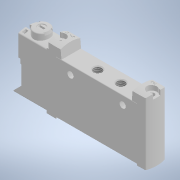
# Autodesk Inventor part: 564212 VUVG-L-10-M52-M-T-M5--1H2--L-W1---(G)
Saved by Autodesk Inventor 2021 (Build 250183000, 183)
## iProperties
Created: 2026-04-25
Part Number: 564212 VUVG-L-10-M52-M-T-M5--1H2--L-W1---(G)
Material: Generic
Catalog Web Link: www.3dfindit.com
Description: VUVG-(G)-Directional control valves for standard applications
Vendor: FESTO
Document SubType Name: Modeling
Designer: psAdmin
Manufacturer: FESTO
Mass: 17.6893 g
Surface Area: 76.999 cm^2
Volume: 17.6893 cm^3
Density: 1 g/cm^3
Appearance: PSOLRGB-176-176-176
Category: PARTsolutions
Company: FESTO
Title: 564212 VUVG-L-10-M52-M-T-M5--1H2--L-W1---(G)
Author: Cadenas PARTsolutions
Comments: Directional control valves for standard applications
PSOL_IDENT_0: {$CADENAS_DATA/23d-libs/festo/parts/v/vuvg/parts/vuvg_gehause.prj},283 {VTYP=3D},{NB=564212 VUVG-L-1
PSOL_IDENT_1: 0-M52-M-T-M5--1H2--L-W1---(G)},{LINA=564212 VUVG-L-10-M52-M-T-M5--1H2--L-W1---(G)},{NN=VUVG-(G)},{DA
PSOL_IDENT_2: TE=05.06.2024 09:23:06},{GEOMDATE=05.06.2024 09:22:54},{VERSION=},{LINEID=10},{WBVAR=VA,KP,BG,VF,RS,
PSOL_IDENT_3: SZ,HHB,PA,EL,NS,EA,SBS,ANZ,EZV,KUP,ZUL},{WBNUMERIC=}  {NB=564212 VUVG-L-10-M52-M-T-M5--1H2--L-W1---(
PSOL_IDENT_4: G)},{LINA=564212 VUVG-L-10-M52-M-T-M5--1H2--L-W1---(G)},{KT=DUMMY},{TNR=564212},{TYP=VUVG},{VA=L},{K
PSOL_IDENT_5: P=-},{BG=10},{VF=M52},{RS=M},{SZ=-},{HHB=T},{PA=M5},{EL=-},{NS=1},{EA=H2},{SBS=-},{ANZ=L},{EZV=W1},{
PSOL_IDENT_6: KUP=-},{ZUL=-},{KZU=-},{L=42},{L1=7.5},{L2=41.62},{H1=1.2},{THREAD=5},{VERS=1},{ASP=1},{CODE=},{SCAL
PSOL_IDENT_7: E=0.5},{ZUL1=},{KZU1=},{ZULT='-'},{KUP1=},{KUPW='-','F1A'}
NB: 564212 VUVG-L-10-M52-M-T-M5--1H2--L-W1---(G)
NN: VUVG-(G)
NT: Directional control valves for standard applications
NBSYN: $TNR. $TYP.-$VA.$KP.$BG.-$VF.-$RS.$SZ.$HHB.-$PA.$EL.-$NS.$EA.-$SBS.$ANZ.-$EZV.$KUP1.$ZUL1.$KZU1.---(G)
LINA: 564212 VUVG-L-10-M52-M-T-M5--1H2--L-W1---(G)
CATALOG: Festo
TNR: 564212
TYP: VUVG
VA: L
KP: -
BG: 10
VF: M52
RS: M
SZ: -
HHB: T
PA: M5
EL: -
NS: 1
EA: H2
SBS: -
ANZ: L
EZV: W1
KUP: -
ZUL: -
KUPW: '-','F1A'
SUPPLIER: FESTO
ARTICLENO: 564212 VUVG-L-10-M52-M-T-M5--1H2--L-W1---(G)
BOMINFO: 564212 VUVG-L-10-M52-M-T-M5--1H2--L-W1---(G)
CREATOR: CADENAS GmbH
Autodesk Inventor part; units mm, degrees
sketch "Sketch_53" plane through (0, 0, 0) normal (1, 0, 0) x (0, 1, 0)
  line L0 (26.7, 5.1) -> (0, 5.1)
  line L1 (0, 5.1) -> (0, -5.1)
  line L2 (0, -5.1) -> (26.7, -5.1)
  arc A0 (26.7, -5.1) -> (27, -4.8) centre (26.7, -4.8) ccw
  line L3 (27, -4.8) -> (27, 4.8)
  arc A1 (27, 4.8) -> (26.7, 5.1) centre (26.7, 4.8) ccw
  constraints: 8 end point, 4 point on circle, 2 centre point
extrude "Extrusion1" add sketch "Sketch_53" along normal mid plane 42
sketch "Sketch_54" plane through (0, 0, 0) normal (0, 0, 1) x (1, 0, 0)
  circle A0 centre (13.5, 22.6) radius 1.6
  constraints: 1 centre point
extrude "Extrusion2" cut sketch "Sketch_54" along normal mid plane 12
sketch "Sketch_55" plane through (0, 0, 0) normal (0, 0, 1) x (1, 0, 0)
  circle A0 centre (-13.5, 22.6) radius 1.6
  constraints: 1 centre point
extrude "Extrusion3" cut sketch "Sketch_55" along normal mid plane 12
sketch "Sketch4" plane through (-21, 0, -5.1) normal (0, -1, 0) x (1, 0, 0)
  point P0 (33.5, 5.1)
hole "Hole1" at (12.5, 0, 0) direction (0, 1, 0) diameter 4.134 depth 13.5 countersink diameter 5 countersink angle 90 thread size "M5x0.8" class "6H" standard "ISO Metric profile"
sketch "Sketch5" plane through (-21, 0, -5.1) normal (0, -1, 0) x (1, 0, 0)
  point P0 (22.5, 5.1)
hole "Hole2" at (1.5, 0, 0) direction (0, 1, 0) diameter 4.134 depth 18.8 tip angle 120 countersink diameter 5 countersink angle 90 thread size "M5x0.8" class "6H" standard "ISO Metric profile"
sketch "Sketch6" plane through (-21, 0, -5.1) normal (0, -1, 0) x (1, 0, 0)
  point P0 (11.5, 5.1)
hole "Hole3" at (-9.5, 0, 0) direction (0, 1, 0) diameter 4.134 depth 13.5 countersink diameter 5 countersink angle 90 thread size "M5x0.8" class "6H" standard "ISO Metric profile"
sketch "Sketch7" plane through (-21, 27, 4.8) normal (0, 1, 0) x (1, 0, 0)
  point P0 (16.5, 4.8)
hole "Hole4" at (-4.5, 27, 0) direction (0, -1, 0) diameter 4.134 depth 6.6 countersink diameter 5 countersink angle 90 thread size "M5x0.8" class "6H" standard "ISO Metric profile"
sketch "Sketch8" plane through (-21, 27, 4.8) normal (0, 1, 0) x (1, 0, 0)
  point P0 (28.5, 4.8)
hole "Hole5" at (7.5, 27, 0) direction (0, -1, 0) diameter 4.134 depth 6.6 countersink diameter 5 countersink angle 90 thread size "M5x0.8" class "6H" standard "ISO Metric profile"
sketch "Sketch9" plane through (7.5, 20.4, 0) normal (0, 1, 0) x (1, 0, 0)
  point P0 (0, 0.495)
hole "Hole6" at (7.5, 20.4, -0.495) direction (0, -1, 0) diameter 3 depth 6.9
sketch "Sketch10" plane through (-4.5, 20.4, 0) normal (0, 1, 0) x (1, 0, 0)
  point P0 (0, -0.505)
hole "Hole7" at (-4.5, 20.4, 0.505) direction (0, -1, 0) diameter 3 depth 6.9
sketch "Sketch_71" plane through (0, -0.8, 0) normal (0, 1, 0) x (1, 0, 0)
  line L0 (21, 5.125) -> (21, -5.125)
  line L1 (21, -5.125) -> (24.9321, -5.0564)
  arc A0 (24.9321, -5.0564) -> (25.3986, -4.712) centre (24.9234, -4.5564) ccw
  arc A1 (25.3986, -4.712) -> (25.3986, 4.712) centre (11, 0) ccw
  arc A2 (25.3986, 4.712) -> (24.9321, 5.0564) centre (24.9234, 4.5564) ccw
  line L2 (24.9321, 5.0564) -> (21, 5.125)
  constraints: 6 end point, 6 point on circle, 3 centre point
extrude "Extrusion4" add sketch "Sketch_71" along normal blind 33.1
sketch "Sketch_20" plane through (0, 27, 0) normal (0, 1, 0) x (1, 0, 0)
  line L0 (18.21, 5.0763) -> (18.21, -5.0763)
  line L1 (18.21, -5.0763) -> (21, -5.125)
  line L2 (21, -5.125) -> (21, 5.125)
  line L3 (21, 5.125) -> (18.21, 5.0763)
  constraints: 8 end point
extrude "Extrusion5" add sketch "Sketch_20" along normal blind 5.7
sketch "Sketch_19" plane through (0, 0, 0) normal (1, 0, 0) x (0, 1, 0)
  arc A0 (31.3973, -5.125) -> (31.3973, 5.125) centre (17.3, 0) ccw
  line L0 (31.3973, -5.125) -> (37, -5.125)
  line L1 (37, -5.125) -> (37, 5.125)
  line L2 (37, 5.125) -> (31.3973, 5.125)
  constraints: 6 end point, 2 point on circle, 1 centre point
sketch "Sketch_22" plane through (0, 0, 0) normal (0, 0, 1) x (1, 0, 0)
  line L0 (13.21, 33) -> (13.21, 27)
  line L1 (13.21, 27) -> (18.21, 27)
  line L2 (18.21, 27) -> (18.7349, 33)
  line L3 (18.7349, 33) -> (13.21, 33)
  constraints: 8 end point
extrude "Extrusion6" cut sketch "Sketch_22" along normal mid plane 12
sketch "Sketch_21" plane through (0, 0, 0) normal (0, 0, 1) x (1, 0, 0)
  line L0 (23.5, -0.8) -> (23.5, 29.7)
  line L1 (23.5, 29.7) -> (24.825, 29.7)
  line L2 (24.825, 29.7) -> (24.625, -0.8)
  line L3 (24.625, -0.8) -> (23.5, -0.8)
  line L4 (23.5, -0.8) -> (23.5, 29.7)
  constraints: 10 end point
revolve "Revolution1" cut sketch "Sketch_21" angle 360 about axis through (23.5, -0.8, 0) along (0, -1, 0)
sketch "Sketch_31" plane through (0, 29.7, 0) normal (0, 1, 0) x (1, 0, 0)
  arc A0 (25.2283, 1.875) -> (25.2283, -1.875) centre (23.5, 0) ccw
  line L0 (25.2283, -1.875) -> (28.5, -1.875)
  line L1 (28.5, -1.875) -> (28.5, 1.875)
  line L2 (28.5, 1.875) -> (25.2283, 1.875)
  constraints: 6 end point, 2 point on circle, 1 centre point
extrude "Extrusion7" cut sketch "Sketch_31" along normal blind 4
sketch "Sketch_32" plane through (0, -0.8, 0) normal (0, 1, 0) x (1, 0, 0)
  line L0 (-25.96, -5.0384) -> (-21, -5.125)
  line L1 (-21, -5.125) -> (-21, 5.125)
  line L2 (-21, 5.125) -> (-25.96, 5.0384)
  line L3 (-25.96, 5.0384) -> (-25.96, -5.0384)
  constraints: 8 end point
extrude "Extrusion8" add sketch "Sketch_32" along normal blind 33.1
sketch "Sketch_33" plane through (0, 27, 0) normal (0, 1, 0) x (1, 0, 0)
  line L0 (-21, -5.125) -> (-18.21, -5.0763)
  line L1 (-18.21, -5.0763) -> (-18.21, 5.0763)
  line L2 (-18.21, 5.0763) -> (-21, 5.125)
  line L3 (-21, 5.125) -> (-21, -5.125)
  constraints: 8 end point
extrude "Extrusion9" add sketch "Sketch_33" along normal blind 5.7
extrude "Extrusion10" cut sketch "Sketch_19" along normal mid plane 64
sketch "Sketch_119" plane through (0, 29.7, 0) normal (0, 1, 0) x (1, 0, 0)
  line L0 (-26.5, -1.875) -> (-25.2283, -1.875)
  arc A0 (-25.2283, -1.875) -> (-25.2283, 1.875) centre (-23.5, 0) ccw
  line L1 (-25.2283, 1.875) -> (-26.5, 1.875)
  line L2 (-26.5, 1.875) -> (-26.5, -1.875)
  constraints: 6 end point, 2 point on circle, 1 centre point
extrude "Extrusion11" cut sketch "Sketch_119" along normal blind 4
sketch "Sketch_36" plane through (0, 0, 0) normal (0, 0, 1) x (1, 0, 0)
  line L0 (-18.7349, 33) -> (-18.21, 27)
  line L1 (-18.21, 27) -> (-13.21, 27)
  line L2 (-13.21, 27) -> (-13.21, 33)
  line L3 (-13.21, 33) -> (-18.7349, 33)
  constraints: 8 end point
extrude "Extrusion12" cut sketch "Sketch_36" along normal mid plane 12
sketch "Sketch_37" plane through (0, 28.5, 0) normal (0, 1, 0) x (1, 0, 0)
  line L0 (-31, -6.125) -> (-21, -6.125)
  line L1 (-21, -6.125) -> (-21, -5.125)
  line L2 (-21, -5.125) -> (-24.7331, -5.0598)
  arc A0 (-25.199, -4.7172) -> (-24.7331, -5.0598) centre (-24.7243, -4.5599) ccw
  arc A1 (-25.199, 4.7172) -> (-25.199, -4.7172) centre (-10.96, 0) ccw
  arc A2 (-24.7331, 5.0598) -> (-25.199, 4.7172) centre (-24.7243, 4.5599) ccw
  line L3 (-24.7331, 5.0598) -> (-21, 5.125)
  line L4 (-21, 5.125) -> (-21, 6.125)
  line L5 (-21, 6.125) -> (-31, 6.125)
  line L6 (-31, 6.125) -> (-31, -6.125)
  constraints: 14 end point, 6 point on circle, 3 centre point
extrude "Extrusion13" cut sketch "Sketch_37" along normal blind 5
sketch "Sketch_38" plane through (-25.96, 0, 0) normal (1, 0, 0) x (0, 0, -1)
  arc A0 (-4.9, 0.7) -> (-4.2, 0) centre (-4.2, 0.7) ccw
  line L0 (-4.2, 0) -> (4.2, 0)
  arc A1 (4.2, 0) -> (4.9, 0.7) centre (4.2, 0.7) ccw
  line L1 (4.9, 0.7) -> (4.9, 27.3163)
  arc A2 (4.9, 27.3163) -> (4.5517, 27.7927) centre (4.4, 27.3163) ccw
  arc A3 (4.5517, 27.7927) -> (-4.5517, 27.7927) centre (0, 13.5) ccw
  arc A4 (-4.5517, 27.7927) -> (-4.9, 27.3163) centre (-4.4, 27.3163) ccw
  line L2 (-4.9, 27.3163) -> (-4.9, 0.7)
  constraints: 10 point on circle, 6 end point, 5 centre point
extrude "Extrusion14" add sketch "Sketch_38" against normal blind 17.2
sketch "Sketch_39" plane through (0, 0, 0) normal (0, 0, 1) x (1, 0, 0)
  line L0 (-43.2, 30) -> (-43.2, 0.7)
  line L1 (-43.2, 0.7) -> (-38.9467, 4.9533)
  line L2 (-38.9467, 4.9533) -> (-38.9467, 16.7)
  line L3 (-38.9467, 16.7) -> (-40.7, 16.7)
  line L4 (-40.7, 16.7) -> (-40.7, 30)
  line L5 (-40.7, 30) -> (-43.2, 30)
  constraints: 12 end point
extrude "Extrusion15" cut sketch "Sketch_39" along normal mid plane 12
sketch "Sketch_40" plane through (0, 13.6, 0) normal (0, 1, 0) x (1, 0, 0)
  line L0 (-40.2, 3.7) -> (-40.2, -3.7)
  arc A0 (-40.2, -3.7) -> (-39.8, -4.1) centre (-39.8, -3.7) ccw
  line L1 (-39.8, -4.1) -> (-38.2, -4.1)
  line L2 (-38.2, -4.1) -> (-38.2, 4.1)
  line L3 (-38.2, 4.1) -> (-39.8, 4.1)
  arc A1 (-39.8, 4.1) -> (-40.2, 3.7) centre (-39.8, 3.7) ccw
  constraints: 8 end point, 4 point on circle, 2 centre point
extrude "Extrusion16" add sketch "Sketch_40" against normal blind 12
sketch "Sketch_41" plane through (0, 13.6, 0) normal (0, 1, 0) x (1, 0, 0)
  line L0 (-40.66, 3.7) -> (-40.66, -3.7)
  arc A0 (-40.66, -3.7) -> (-40.26, -4.1) centre (-40.26, -3.7) ccw
  line L1 (-40.26, -4.1) -> (-37.66, -4.1)
  line L2 (-37.66, -4.1) -> (-37.66, 4.1)
  line L3 (-37.66, 4.1) -> (-40.26, 4.1)
  arc A1 (-40.26, 4.1) -> (-40.66, 3.7) centre (-40.26, 3.7) ccw
  constraints: 8 end point, 4 point on circle, 2 centre point
extrude "Extrusion17" add sketch "Sketch_41" along normal blind 3.1
sketch "Sketch_42" plane through (-40.2, 0, 0) normal (1, 0, 0) x (0, 0, -1)
  line L0 (-3.45, 11.8) -> (-3.45, 0)
  line L1 (-3.45, 0) -> (3.45, 0)
  line L2 (3.45, 0) -> (3.45, 11.8)
  arc A0 (3.45, 11.8) -> (2.65, 12.6) centre (2.65, 11.8) ccw
  line L3 (2.65, 12.6) -> (-2.65, 12.6)
  arc A1 (-2.65, 12.6) -> (-3.45, 11.8) centre (-2.65, 11.8) ccw
  constraints: 8 end point, 4 point on circle, 2 centre point
extrude "Extrusion18" add sketch "Sketch_42" against normal blind 0.1
sketch "Sketch_43" plane through (-40.2, 0, 0) normal (1, 0, 0) x (0, 0, -1)
  arc A0 (-2.85, 4.7) -> (-2.35, 4.2) centre (-2.35, 4.7) ccw
  line L0 (-2.35, 4.2) -> (2.35, 4.2)
  arc A1 (2.35, 4.2) -> (2.85, 4.7) centre (2.35, 4.7) ccw
  line L1 (2.85, 4.7) -> (2.85, 11.5)
  arc A2 (2.85, 11.5) -> (2.35, 12) centre (2.35, 11.5) ccw
  line L2 (2.35, 12) -> (-2.35, 12)
  arc A3 (-2.35, 12) -> (-2.85, 11.5) centre (-2.35, 11.5) ccw
  line L3 (-2.85, 11.5) -> (-2.85, 4.7)
  constraints: 8 end point, 8 point on circle, 4 centre point
extrude "Extrusion19" cut sketch "Sketch_43" along normal mid plane 1
sketch "Sketch_44" plane through (0, 9.65, 0) normal (0, 1, 0) x (1, 0, 0)
  line L0 (-40.85, -1.25) -> (-40.85, -1.75)
  line L1 (-40.85, -1.75) -> (-35.85, -1.75)
  line L2 (-35.85, -1.75) -> (-35.85, 1.75)
  line L3 (-35.85, 1.75) -> (-40.85, 1.75)
  line L4 (-40.85, 1.75) -> (-40.85, 1.25)
  line L5 (-40.85, 1.25) -> (-36.35, 1.25)
  line L6 (-36.35, 1.25) -> (-36.35, -1.25)
  line L7 (-36.35, -1.25) -> (-40.85, -1.25)
  constraints: 16 end point
extrude "Extrusion20" add sketch "Sketch_44" against normal blind 2.6
sketch "Sketch_34" plane through (0, 0, 0) normal (0, 0, 1) x (1, 0, 0)
  line L0 (-23.5, -0.8) -> (-23.5, 29.7)
  line L1 (-23.5, 29.7) -> (-22.175, 29.7)
  line L2 (-22.175, 29.7) -> (-22.375, -0.8)
  line L3 (-22.375, -0.8) -> (-23.5, -0.8)
  line L4 (-23.5, -0.8) -> (-23.5, 29.7)
  constraints: 10 end point
revolve "Revolution2" cut sketch "Sketch_34" angle 360 about axis through (-23.5, -0.8, 0) along (0, -1, 0)
sketch "Sketch_61" plane through (0, 0, 0) normal (0, 0, 1) x (1, 0, 0)
  line L0 (-33.46, 26.365) -> (-33.46, 31.665)
  line L1 (-33.46, 31.665) -> (-29.41, 31.665)
  line L2 (-29.41, 31.665) -> (-29.41, 26.365)
  line L3 (-29.41, 26.365) -> (-33.46, 26.365)
  line L4 (-33.46, 26.365) -> (-33.46, 31.665)
  constraints: 10 end point
revolve "Revolution3" add sketch "Sketch_61" angle 360 about axis through (-33.46, 26.365, 0) along (0, -1, 0)
sketch "Sketch_62" plane through (0, 30.1, 0) normal (0, 1, 0) x (1, 0, 0)
  circle A0 centre (-33.46, 0) radius 6
  arc A1 (-38.0426, -2) -> (-28.8774, -2) centre (-33.46, 0) ccw
  line L0 (-28.8774, -2) -> (-30.7105, -2)
  arc A2 (-30.7105, -2) -> (-30.7105, 2) centre (-33.46, 0) ccw
  line L1 (-30.7105, 2) -> (-28.8774, 2)
  arc A3 (-28.8774, 2) -> (-38.0426, 2) centre (-33.46, 0) ccw
  line L2 (-38.0426, 2) -> (-36.2095, 2)
  arc A4 (-36.2095, 2) -> (-36.2095, -2) centre (-33.46, 0) ccw
  line L3 (-36.2095, -2) -> (-38.0426, -2)
  constraints: 8 end point, 8 point on circle, 5 centre point
extrude "Extrusion21" cut sketch "Sketch_62" along normal blind 3
sketch "Sketch_63" plane through (0, 0, 0) normal (0, 0, 1) x (1, 0, 0)
  line L0 (-33.46, 26.365) -> (-33.46, 31.665)
  line L1 (-30.06, 31.4408) -> (-30.06, 26.365)
  line L2 (-30.06, 26.365) -> (-29.41, 26.365)
  line L3 (-29.41, 26.365) -> (-29.41, 29.115)
  line L4 (-29.41, 29.115) -> (-29.81, 29.115)
  line L5 (-29.81, 29.115) -> (-29.81, 30.015)
  line L6 (-29.81, 30.015) -> (-29.41, 30.015)
  line L7 (-29.41, 30.015) -> (-29.41, 30.315)
  line L8 (-29.41, 30.315) -> (-30.06, 31.4408)
  constraints: 18 end point
revolve "Revolution4" add sketch "Sketch_63" angle 360 about axis through (-33.46, 26.365, 0) along (0, -1, 0)
sketch "Sketch_64" plane through (0, 0, 0) normal (0, 0, 1) x (1, 0, 0)
  line L0 (-33.46, 30.295) -> (-33.46, 32.365)
  line L1 (-33.46, 32.365) -> (-28.46, 32.365)
  line L2 (-28.46, 32.365) -> (-28.46, 28.865)
  line L3 (-28.46, 28.865) -> (-29.41, 28.865)
  line L4 (-29.41, 28.865) -> (-29.41, 30.9614)
  arc A0 (-29.41, 30.9614) -> (-29.71, 31.3487) centre (-29.81, 30.9614) ccw
  arc A1 (-29.71, 31.3487) -> (-31.2809, 31.6659) centre (-33.46, 16.825) ccw
  arc A2 (-31.2809, 31.6659) -> (-31.51, 31.468) centre (-31.31, 31.468) ccw
  line L5 (-31.51, 31.468) -> (-31.51, 30.295)
  line L6 (-31.51, 30.295) -> (-33.46, 30.295)
  line L7 (-33.46, 30.295) -> (-33.46, 32.365)
  constraints: 16 end point, 6 point on circle, 3 centre point
revolve "Revolution5" cut sketch "Sketch_64" angle 360 about axis through (-33.46, 30.295, 0) along (0, -1, 0)
sketch "Sketch_65" plane through (0, 0, 0) normal (0, 0, 1) x (1, 0, 0)
  line L0 (-33.46, 25.41) -> (-33.46, 31.41)
  line L1 (-33.46, 31.41) -> (-31.9158, 31.41)
  line L2 (-31.9158, 31.41) -> (-31.56, 31.36)
  line L3 (-31.56, 31.36) -> (-31.56, 29.71)
  arc A0 (-31.56, 29.71) -> (-31.06, 29.21) centre (-31.06, 29.71) ccw
  line L4 (-31.06, 29.21) -> (-30.91, 29.21)
  line L5 (-30.91, 29.21) -> (-30.91, 25.41)
  line L6 (-30.91, 25.41) -> (-33.46, 25.41)
  line L7 (-33.46, 25.41) -> (-33.46, 31.41)
  constraints: 16 end point, 2 point on circle, 1 centre point
revolve "Revolution6" add sketch "Sketch_65" angle 360 about axis through (-33.46, 25.41, 0) along (0, -1, 0)
sketch "Sketch_66" plane through (0, 31.41, 0) normal (0, 1, 0) x (1, 0, 0)
  arc A0 (-34.853, 0.5) -> (-34.853, -0.5) centre (-33.46, 0) ccw
  line L0 (-34.853, -0.5) -> (-32.067, -0.5)
  arc A1 (-32.067, -0.5) -> (-32.067, 0.5) centre (-33.46, 0) ccw
  line L1 (-32.067, 0.5) -> (-34.853, 0.5)
  constraints: 4 end point, 4 point on circle, 2 centre point
extrude "Extrusion22" cut sketch "Sketch_66" against normal blind 2.15
sketch "Sketch_82" plane through (0, 0, 0) normal (0, 0, 1) x (1, 0, 0)
  line L0 (-43.16, 4.2) -> (-43.16, 0.2)
  line L1 (-43.16, 0.2) -> (-42.16, 1.2)
  line L2 (-42.16, 1.2) -> (-40.66, 1.2)
  line L3 (-40.66, 1.2) -> (-40.66, 4.2)
  line L4 (-40.66, 4.2) -> (-43.16, 4.2)
  constraints: 10 end point
extrude "Extrusion23" cut sketch "Sketch_82" along normal mid plane 7.8
sketch "Sketch_81" plane through (0, 0, 0) normal (0, 0, 1) x (1, 0, 0)
  line L0 (-45.756, 28.534) -> (-45.756, 17.4808)
  line L1 (-45.756, 17.4808) -> (-38.256, 23.774)
  line L2 (-38.256, 23.774) -> (-38.256, 28.534)
  line L3 (-38.256, 28.534) -> (-45.756, 28.534)
  constraints: 8 end point
extrude "Extrusion24" cut sketch "Sketch_81" along normal mid plane 2.1
sketch "Sketch_85" plane through (0, 0, 0) normal (0, 0, 1) x (1, 0, 0)
  line L0 (-45.9, 1.9535) -> (-45.9, 1.2004)
  line L1 (-45.9, 1.2004) -> (-41.9479, 1.0624)
  arc A0 (-41.8553, 0.9349) -> (-41.9479, 1.0624) centre (-41.9514, 0.9625) ccw
  line L2 (-41.8553, 0.9349) -> (-41.9956, 0.4457)
  arc A1 (-41.9956, 0.4457) -> (-41.9012, 0.3181) centre (-41.8994, 0.4181) ccw
  line L3 (-41.9012, 0.3181) -> (-41.7605, 0.3157)
  arc A2 (-41.7605, 0.3157) -> (-41.5443, 0.412) centre (-41.7557, 0.5957) ccw
  line L4 (-41.5443, 0.412) -> (-41.0599, 0.9693)
  arc A3 (-41.0599, 0.9693) -> (-41.4198, 1.797) centre (-41.4372, 1.2973) ccw
  line L5 (-41.4198, 1.797) -> (-45.9, 1.9535)
  constraints: 12 end point, 8 point on circle, 4 centre point
extrude "Extrusion25" cut sketch "Sketch_85" along normal mid plane 7.8
sketch "Sketch_94" plane through (-43.2, 0, 0) normal (1, 0, 0) x (0, 0, -1)
  line L0 (-4.25, 13.012) -> (4.25, 13.012)
  line L1 (4.25, 13.012) -> (4.25, 27.012)
  line L2 (4.25, 27.012) -> (-4.25, 27.012)
  line L3 (-4.25, 27.012) -> (-4.25, 13.012)
  constraints: 8 end point
extrude "Extrusion26" cut sketch "Sketch_94" along normal blind 2.8
sketch "Sketch_133" plane through (-38.36, 0, 0) normal (1, 0, 0) x (0, 0, -1)
  line L0 (-3.9, 31) -> (-3.9, 25)
  line L1 (-3.9, 25) -> (-2, 25)
  line L2 (-2, 25) -> (-2, 30)
  line L3 (-2, 30) -> (2, 30)
  line L4 (2, 30) -> (2, 25)
  line L5 (2, 25) -> (3.9, 25)
  line L6 (3.9, 25) -> (3.9, 31)
  line L7 (3.9, 31) -> (-3.9, 31)
  constraints: 16 end point
extrude "Extrusion27" cut sketch "Sketch_133" against normal blind 1.5
sketch "Sketch_136" plane through (-38.36, 0, 0) normal (1, 0, 0) x (0, 0, -1)
  line L0 (-3.9, 27) -> (-3.9, 24)
  line L1 (-3.9, 24) -> (-2, 24)
  line L2 (-2, 24) -> (-2, 27)
  line L3 (-2, 27) -> (-3.9, 27)
  constraints: 8 end point
extrude "Extrusion28" cut sketch "Sketch_136" against normal blind 3
sketch "Sketch_137" plane through (-38.36, 0, 0) normal (1, 0, 0) x (0, 0, -1)
  line L0 (2, 27) -> (2, 24)
  line L1 (2, 24) -> (3.9, 24)
  line L2 (3.9, 24) -> (3.9, 27)
  line L3 (3.9, 27) -> (2, 27)
  constraints: 8 end point
extrude "Extrusion29" cut sketch "Sketch_137" against normal blind 3
sketch "Sketch_12" plane through (0, 31.7, 0) normal (0, 1, 0) x (1, 0, 0)
  line L0 (-24.6, 3.175) -> (-24.138, 2.8515)
  line L1 (-24.138, 2.8515) -> (-24.0676, 2.9522)
  line L2 (-24.0676, 2.9522) -> (-24.3858, 3.175)
  line L3 (-24.3858, 3.175) -> (-23.55, 3.175)
  line L4 (-23.55, 3.175) -> (-23.55, 2.875)
  line L5 (-23.55, 2.875) -> (-23.4, 2.875)
  line L6 (-23.4, 2.875) -> (-23.4, 3.625)
  line L7 (-23.4, 3.625) -> (-23.55, 3.625)
  line L8 (-23.55, 3.625) -> (-23.55, 3.325)
  line L9 (-23.55, 3.325) -> (-24.6, 3.325)
  line L10 (-24.6, 3.325) -> (-24.6, 3.175)
  constraints: 22 end point
extrude "Extrusion30" cut sketch "Sketch_12" along normal mid plane 2
sketch "Sketch_68" plane through (0, 31.7, 0) normal (0, 1, 0) x (1, 0, 0)
  line L0 (-24.6, 4.2508) -> (-23.7083, 3.835)
  line L1 (-23.7083, 3.835) -> (-23.6, 3.835)
  line L2 (-23.6, 3.835) -> (-23.6, 4.25)
  line L3 (-23.6, 4.25) -> (-23.4, 4.25)
  line L4 (-23.4, 4.25) -> (-23.4, 4.4)
  line L5 (-23.4, 4.4) -> (-23.6, 4.4)
  line L6 (-23.6, 4.4) -> (-23.6, 4.665)
  line L7 (-23.6, 4.665) -> (-23.75, 4.665)
  line L8 (-23.75, 4.665) -> (-23.75, 4.4)
  line L9 (-23.75, 4.4) -> (-23.9, 4.4)
  line L10 (-23.9, 4.4) -> (-23.9, 4.25)
  line L11 (-23.9, 4.25) -> (-23.75, 4.25)
  line L12 (-23.75, 4.25) -> (-23.75, 4.0199)
  line L13 (-23.75, 4.0199) -> (-24.6, 4.4163)
  line L14 (-24.6, 4.4163) -> (-24.6, 4.2508)
  constraints: 30 end point
extrude "Extrusion31" cut sketch "Sketch_68" along normal mid plane 2
sketch "Sketch_101" plane through (0, 31.7, 0) normal (0, 1, 0) x (1, 0, 0)
  line L0 (-22.4, 3.5016) -> (-20.6166, 2.67)
  line L1 (-20.6166, 2.67) -> (-20.4, 2.67)
  line L2 (-20.4, 2.67) -> (-20.4, 3.5)
  line L3 (-20.4, 3.5) -> (-20, 3.5)
  line L4 (-20, 3.5) -> (-20, 3.8)
  line L5 (-20, 3.8) -> (-20.4, 3.8)
  line L6 (-20.4, 3.8) -> (-20.4, 4.33)
  line L7 (-20.4, 4.33) -> (-20.7, 4.33)
  line L8 (-20.7, 4.33) -> (-20.7, 3.8)
  line L9 (-20.7, 3.8) -> (-21, 3.8)
  line L10 (-21, 3.8) -> (-21, 3.5)
  line L11 (-21, 3.5) -> (-20.7, 3.5)
  line L12 (-20.7, 3.5) -> (-20.7, 3.0399)
  line L13 (-20.7, 3.0399) -> (-22.4, 3.8326)
  line L14 (-22.4, 3.8326) -> (-22.4, 3.5016)
  constraints: 30 end point
extrude "Extrusion32" cut sketch "Sketch_101" along normal mid plane 2
sketch "Sketch_102" plane through (0, 31.7, 0) normal (0, 1, 0) x (1, 0, 0)
  arc A0 (20.8536, 3.9962) -> (20.325, 2.775) centre (20.325, 3.5) ccw
  line L0 (20.325, 2.775) -> (20.325, 3.075)
  arc A1 (20.6349, 3.7909) -> (20.325, 3.075) centre (20.325, 3.5) ccw
  line L1 (20.6349, 3.7909) -> (21.5885, 2.775)
  line L2 (21.5885, 2.775) -> (22, 2.775)
  line L3 (22, 2.775) -> (22, 4.225)
  line L4 (22, 4.225) -> (21.7, 4.225)
  line L5 (21.7, 4.225) -> (21.7, 3.0946)
  line L6 (21.7, 3.0946) -> (20.8536, 3.9962)
  constraints: 14 end point, 4 point on circle, 2 centre point
extrude "Extrusion33" cut sketch "Sketch_102" along normal mid plane 2
ref_plane "DICHTUNG_XY" through (1.5, 0, 0) normal (0, 1, 0) x (1, 0, 0)
ref_plane "DICHTUNG_YZ" through (1.5, 0, 0) normal (1, 0, 0) x (0, 0, -1)
ref_plane "DICHTUNG_ZX" through (1.5, 0, 0) normal (0, 0, -1) x (0, 1, 0)
ref_plane "GEHAUSE_XY" through (0, 0, 0) normal (0, 1, 0) x (1, 0, 0)
ref_plane "GEHAUSE_YZ" through (0, 0, 0) normal (1, 0, 0) x (0, 0, -1)
ref_plane "GEHAUSE_ZX" through (0, 0, 0) normal (0, 0, -1) x (0, 1, 0)
ref_plane "HHB2_XY" through (-33.46, 31.66, 0) normal (0, 1, 0) x (1, 0, 0)
ref_plane "HHB2_YZ" through (-33.46, 31.66, 0) normal (1, 0, 0) x (0, 0, -1)
ref_plane "HHB2_ZX" through (-33.46, 31.66, 0) normal (0, 0, -1) x (0, 1, 0)
ref_plane "NEBV2_XY" through (-45.896, 24.712, 0) normal (-1, 0, 0) x (0, 0, -1)
ref_plane "NEBV2_YZ" through (-45.896, 24.712, 0) normal (0, 0, -1) x (0, -1, 0)
ref_plane "NEBV2_ZX" through (-45.896, 24.712, 0) normal (0, -1, 0) x (-1, 0, 0)
ref_plane "QS_K1_XY" through (1.5, 0, 0) normal (0, 1, 0) x (1, 0, 0)
ref_plane "QS_K1_YZ" through (1.5, 0, 0) normal (1, 0, 0) x (0, 0, -1)
ref_plane "QS_K1_ZX" through (1.5, 0, 0) normal (0, 0, -1) x (0, 1, 0)
ref_plane "QS_K1214_XY" through (-14.2, 27, -1.605) normal (0, -1, 0) x (1, 0, 0)
ref_plane "QS_K1214_YZ" through (-14.2, 27, -1.605) normal (1, 0, 0) x (0, 0, 1)
ref_plane "QS_K1214_ZX" through (-14.2, 27, -1.605) normal (0, 0, 1) x (0, -1, 0)
ref_plane "QS_K2_XY" through (7.5, 27, 0) normal (0, -1, 0) x (1, 0, 0)
ref_plane "QS_K2_YZ" through (7.5, 27, 0) normal (1, 0, 0) x (0, 0, 1)
ref_plane "QS_K2_ZX" through (7.5, 27, 0) normal (0, 0, 1) x (0, -1, 0)
ref_plane "QS_K3_XY" through (12.5, 0, 0) normal (0, 1, 0) x (1, 0, 0)
ref_plane "QS_K3_YZ" through (12.5, 0, 0) normal (1, 0, 0) x (0, 0, -1)
ref_plane "QS_K3_ZX" through (12.5, 0, 0) normal (0, 0, -1) x (0, 1, 0)
ref_plane "QS_K4_XY" through (-4.5, 27, 0) normal (0, -1, 0) x (1, 0, 0)
ref_plane "QS_K4_YZ" through (-4.5, 27, 0) normal (1, 0, 0) x (0, 0, 1)
ref_plane "QS_K4_ZX" through (-4.5, 27, 0) normal (0, 0, 1) x (0, -1, 0)
ref_plane "QS_K5_XY" through (-9.5, 0, 0) normal (0, 1, 0) x (1, 0, 0)
ref_plane "QS_K5_YZ" through (-9.5, 0, 0) normal (1, 0, 0) x (0, 0, -1)
ref_plane "QS_K5_ZX" through (-9.5, 0, 0) normal (0, 0, -1) x (0, 1, 0)
ref_plane "SCREW1_XY" through (23.5, 29.7, 0) normal (0, 1, 0) x (1, 0, 0)
ref_plane "SCREW1_YZ" through (23.5, 29.7, 0) normal (1, 0, 0) x (0, 0, -1)
ref_plane "SCREW1_ZX" through (23.5, 29.7, 0) normal (0, 0, -1) x (0, 1, 0)
ref_plane "SCREW2_XY" through (-23.5, 29.7, 0) normal (0, 1, 0) x (1, 0, 0)
ref_plane "SCREW2_YZ" through (-23.5, 29.7, 0) normal (1, 0, 0) x (0, 0, -1)
ref_plane "SCREW2_ZX" through (-23.5, 29.7, 0) normal (0, 0, -1) x (0, 1, 0)
ref_plane "VAVE1_XY" through (-41.62, 1.2, 0) normal (0, 1, 0) x (1, 0, 0)
ref_plane "VAVE1_YZ" through (-41.62, 1.2, 0) normal (1, 0, 0) x (0, 0, -1)
ref_plane "VAVE1_ZX" through (-41.62, 1.2, 0) normal (0, 0, -1) x (0, 1, 0)
body "Solid1"
